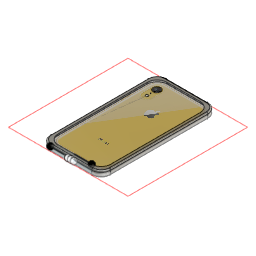
phoneCase v1 (Autodesk Fusion 360 design; units mm, degrees)
Autodesk Fusion 360 part; units mm, degrees
sketch "Sketch1" plane through (0, 0, 0) normal (0, 0, 1) x (1, 0, 0)
  line L0 (0, 0) -> (155.956, 0)
  line L1 (155.956, 0) -> (155.956, 80.772)
  line L2 (155.956, 80.772) -> (0, 80.772)
  line L3 (0, 80.772) -> (0, 0)
  dimension "d1" = 155.956
  dimension "d2" = 80.772
  constraint horizontal L0
  constraint vertical L1
  constraint horizontal L2
  constraint vertical L3
  constraint coincident L0.start L3.end
  measures "d1" distance of L0.start L0.end
  measures "d2" distance of L0.start L2.end
sketch "Sketch2" plane through (0, 0, 0) normal (0, 0, 1) x (1, 0, 0)
  line L0 (0, 0) -> (80.772, 0)
  line L1 (80.772, 0) -> (80.772, 155.956)
  line L2 (80.772, 155.956) -> (0, 155.956)
  line L3 (0, 155.956) -> (0, 0)
  dimension "d8" = 80.772
  dimension "d9" = 155.956
  constraint horizontal L0
  constraint vertical L1
  constraint horizontal L2
  constraint vertical L3
  constraint coincident L0.start L3.end
  measures "d8" distance of L0.start L0.end
  measures "d9" distance of L0.start L2.end
extrude "Extrude2" add sketch "Sketch2" along normal blind 8.382
shell "Shell2" thickness 5.08 removed faces 1 at (26.924, 103.9707, 8.382)
fillet "Fillet2" radius 12.7 4 edges at (5.08, 150.876, 6.731) (75.692, 150.876, 6.731) (75.692, 5.08, 6.731) (5.08, 5.08, 6.731)
sketch "Sketch3" plane through (0, 0, 0) normal (0, 0, -1) x (1, 0, 0)
  line L0 (0, 0) -> (0, -155.956)
  line L1 (0, -155.956) -> (80.772, -155.956)
  line L2 (80.772, -155.956) -> (80.772, 0)
  line L3 (80.772, 0) -> (0, 0)
  circle A0 centre (16.8165, -138.7849) radius 4.9817
  circle A1 centre (16.8165, -130.4826) radius 0.5236
  circle A2 centre (16.8165, -125.4712) radius 1.8106
extrude "Extrude3" cut sketch "Sketch3" against normal blind 6.35 contours A0 | A1 | A2
fillet "Fillet3" radius 12.7 4 edges at (0, 155.956, 4.191) (0, 0, 4.191) (80.772, 155.956, 4.191) (80.772, 0, 4.191)
fillet "Fillet4" radius 1.778 16 edges at (77.0523, 152.2363, 8.382) (40.386, 155.956, 8.382) (3.7197, 152.2363, 8.382) (0, 77.978, 8.382) (3.7197, 3.7197, 8.382) (40.386, 0, 8.382) (77.0523, 3.7197, 8.382) (80.772, 77.978, 8.382) (3.7197, 152.2363, 0) (0, 77.978, 0) (3.7197, 3.7197, 0) (40.386, 0, 0) (77.0523, 3.7197, 0) (80.772, 77.978, 0) (77.0523, 152.2363, 0) (40.386, 155.956, 0)
draft "Draft1" angle -20 neutral plane through (0, 0, 8.382) pull (0, 0, 1) 8 faces at (75.692, 57.912, 7.2813) (63.5963, 5.0944, 7.2813) (32.8507, 5.08, 6.1807) (17.1757, 5.0944, 6.1807) (5.08, 98.044, 7.2813) (17.1757, 150.8616, 7.2813) (32.8507, 150.876, 7.2813) (68.8115, 149.4642, 7.2813)
sketch "Sketch5" plane through (0, 1.7918, -0.6522) normal (0, 0.939693, -0.34202) x (-1, 0, 0)
  line L0 (-17.78, 6.1001) -> (-17.78, 9.614)
  line L1 (-17.78, 9.614) -> (-62.992, 9.614)
  line L2 (-62.992, 9.614) -> (-62.992, 6.1001)
  line L3 (-62.992, 6.1001) -> (-17.78, 6.1001)
  line L4 (-62.992, 9.614) -> (-40.386, 9.614)
  constraint coincident L1.end L2.start
  constraint midpoint L1 L4.end
sketch "Sketch6" plane through (0, 0, 0) normal (0, -1, 0) x (1, 0, 0)
  line L0 (12.7, 1.778) -> (68.072, 1.778)
  line L1 (68.072, 1.778) -> (68.072, 6.604)
  line L2 (68.072, 6.604) -> (12.7, 6.604)
  line L3 (12.7, 6.604) -> (12.7, 1.778)
  line L4 (12.7, 6.604) -> (40.386, 6.604)
  line L5 (40.386, 5.1735) -> (36.576, 5.1735)
  line L6 (40.386, 5.1735) -> (36.576, 5.1735)
  line L7 (40.386, 5.1735) -> (44.196, 5.1735)
  dimension "d24" = 3.81
  dimension "d25" = 3.81
  dimension "d26" = 3.81
  constraint coincident L2.end L3.start
  constraint midpoint L2 L4.end
  constraint perpendicular L3 L5
  constraint parallel L5 L7
  measures "d24" distance of L5.start L5.end
  measures "d25" distance of L5.end L5.start
  measures "d26" distance of L5.start L7.end
draft "Draft2" angle 25 neutral plane through (0, 0, 8.382) pull (0, 0, 1) 8 faces at (76.0926, 98.044, 7.2813) (67.4078, 5.0213, 6.1807) (47.9213, 4.6794, 7.2813) (5.2459, 12.7621, 6.1807) (4.2788, 98.044, 6.1807) (6.0876, 144.9266, 6.1807) (32.8507, 151.2766, 7.2813) (70.8235, 149.1738, 6.1807)
draft "Draft3" angle -30 neutral plane through (0, 0, 8.382) pull (0, 0, 1) 8 faces at (75.5957, 57.912, 7.2813) (68.7674, 6.5774, 7.2813) (47.9213, 5.2726, 6.1807) (7.8728, 9.9889, 7.2813) (5.2726, 57.912, 6.1807) (7.5133, 145.4869, 7.2813) (47.9213, 150.7797, 7.2813) (68.7674, 149.3786, 7.2813)
